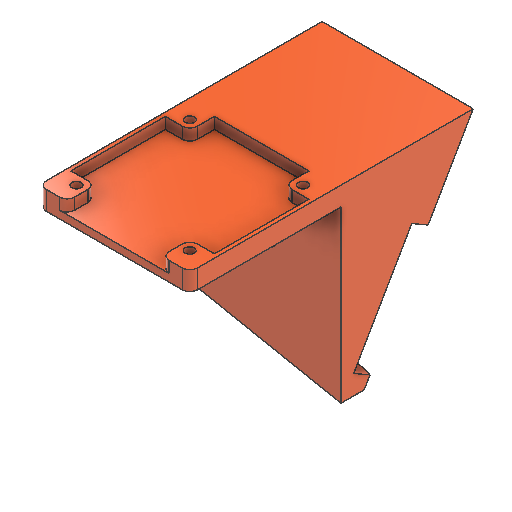
# Autodesk Inventor part: CameraMountM12v2
Saved by Autodesk Inventor 2025.2 (Build 292293000, 293)
## iProperties
Created: 2024-07-04
Part Number: CameraMountM12v2
Material: Generic
Document SubType Name: Modeling
Designer: rolan
Density: 1 g/cm^3
Appearance: Default
Author: rolan
Autodesk Inventor part; units mm, degrees
ref_plane "YZ Plane" through (0, 0, 0) normal (1, 0, 0) x (0, 1, 0)
ref_plane "XZ Plane" through (0, 0, 0) normal (0, 1, 0) x (-1, 0, 0)
sketch "Sketch1" plane through (0, 0, 0) normal (0, 1, 0) x (-1, 0, 0)
  line L0 (19, 19) -> (-19, 19) construction
  line L1 (-19, 19) -> (-19, -19) construction
  line L2 (-19, -19) -> (19, -19) construction
  line L3 (19, -19) -> (19, 19) construction
  line L4 (19, 19) -> (-19, -19) construction
  line L5 (-19, 19) -> (19, -19) construction
  circle A0 centre (15, -15) radius 1.25
  circle A1 centre (-15, -15) radius 1.25
  circle A2 centre (15, 15) radius 1.25
  circle A3 centre (-15, 15) radius 1.25
  line L6 (20, 20) -> (-20, 20)
  line L7 (-20, 20) -> (-20, -20)
  line L8 (-20, -20) -> (20, -20)
  line L9 (20, -20) -> (20, 20)
  line L10 (20, 20) -> (-20, -20) construction
  line L11 (-20, 20) -> (20, -20) construction
  point P0 (0, 0)
  dimension "d0" = 38
  dimension "d1" = 38
  dimension "d2" = 2.5
  dimension "d3" = 2.5
  dimension "d4" = 2.5
  dimension "d5" = 2.5
  dimension "d6" = 4
  dimension "d7" = 4
  dimension "d8" = 4
  dimension "d9" = 4
  dimension "d10" = 40
  dimension "d11" = 40
  constraints: 24 end point, 4 centre point, 4 midpoint, 4 parallel, 2 horizontal, 2 horizontal alignment, 2 perpendicular, 2 vertical alignment
  measures "d0" distance of L1.end L2.end
  measures "d1" distance of L0.end L1.end
  measures "d2" diameter of A1
  measures "d3" diameter of A0
  measures "d4" diameter of A2
  measures "d5" diameter of A3
  measures "d6" distance from line of L2 A0.centre
  measures "d7" distance from line of L3 A0.centre
  measures "d8" distance from line of L0 A3.centre
  measures "d9" distance from line of L1 A3.centre
  measures "d10" distance of L8.end L7.end
  measures "d11" distance of L7.end L6.end
extrude "Extrusion1" add sketch "Sketch1" along normal blind 5
sketch "Sketch2" plane through (0, 5, 0) normal (0, 1, 0) x (1, 0, 0)
  line L0 (-12.5, 19) -> (-12.5, 12.5)
  line L1 (-12.5, 12.5) -> (-19, 12.5)
  line L2 (-19, 12.5) -> (-19, -12.5)
  line L3 (-20, 20) -> (-20, -20) projected
  line L4 (-19, -12.5) -> (-12.5, -12.5)
  line L5 (-12.5, -12.5) -> (-12.5, -20)
  line L6 (-12.5, -20) -> (12.5, -20)
  line L7 (12.5, -20) -> (12.5, -12.5)
  line L8 (12.5, -12.5) -> (19, -12.5)
  line L9 (19, -12.5) -> (19, 12.5)
  line L10 (19, 12.5) -> (12.5, 12.5)
  line L11 (12.5, 12.5) -> (12.5, 19)
  line L12 (12.5, 19) -> (-12.5, 19)
  point P0 (0, 0)
  dimension "d14" = 25
  dimension "d15" = 6.5
  dimension "d16" = 25
  dimension "d17" = 7.5
  dimension "d18" = 6.5
  dimension "d19" = 6.5
  dimension "d20" = 25
  dimension "d21" = 6.5
  dimension "d22" = 12.5
  dimension "d24" = 12.5
  constraints: 24 end point, 8 perpendicular, 4 point on line, 1 parallel, 1 vertical
  measures "d14" distance of L0.start L11.end
  measures "d15" distance of L10.end L11.end
  measures "d16" distance of L8.end L9.end
  measures "d17" distance between parallel lines of L6 L8
  measures "d18" distance between parallel lines of L9 L11
  measures "d19" distance between parallel lines of L9 L7
  measures "d20" distance of L5.end L6.end
  measures "d21" distance between parallel lines of L2 L5
  measures "d22" horizontal distance of point (0, 0) L0.start
  measures "d24" horizontal distance of point (0, 0) L0.end
extrude "Extrusion2" cut sketch "Sketch2" against normal blind 3
sketch "Sketch3" plane through (0, 2, 0) normal (0, 1, 0) x (1, 0, 0)
  line L0 (12.5, -12.5) -> (12.5, -20) projected
  line L1 (-12.5, -20) -> (12.5, -20)
  line L2 (12.5, -20) -> (12.5, -16)
  line L3 (12.5, -16) -> (-12.5, -16)
  line L4 (-12.5, -16) -> (-12.5, -20)
  point P0 (0, 0)
  dimension "d27" = 4
  constraints: 8 end point, 2 parallel, 1 horizontal, 1 perpendicular, 1 point on line
  measures "d27" distance of L2.end L1.end
extrude "Extrusion3" cut sketch "Sketch3" against normal through all
fillet "Fillet1" radius 2 10 edges at (-20, 2.5, -20) (20, 2.5, -20) (-20, 2.5, 20) (20, 2.5, 20) (-12.5, 3.5, -12.5) (12.5, 3.5, -12.5) (12.5, 3.5, 12.5) (-12.5, 3.5, 12.5) (-12.5, 2.5, 20) (12.5, 2.5, 20)
sketch "Sketch4" plane through (0, 0, 0) normal (0, -1, 0) x (1, 0, 0)
  line L0 (-20, -17.5) -> (20, -17.5)
  line L1 (20, -17.5) -> (20, 17.5)
  line L2 (20, 17.5) -> (-20, 17.5)
  line L3 (-20, 17.5) -> (-20, -17.5)
  line L4 (-20, -17.5) -> (20, 17.5) construction
  line L5 (20, -17.5) -> (-20, 17.5) construction
  point P0 (0, 0)
  dimension "d31" = 40
  dimension "d32" = 35
  constraints: 12 end point, 2 midpoint, 2 parallel, 1 horizontal, 1 perpendicular
  measures "d31" distance of L2.end L1.end
  measures "d32" distance of L1.end L0.end
extrude "Extrusion4" add sketch "Sketch4" along normal blind 50
sketch "Sketch6" plane through (-20, 0, 17.5) normal (0, 0, 1) x (1, 0, 0)
  line L0 (40, 0) -> (40, -50) projected
  line L1 (40, -50) -> (0, -42.0435)
  line L2 (0, 0) -> (0, -50) projected
  line L3 (40, -50) -> (80.7836, -50) construction
  line L4 (0, -42.0435) -> (0, -50)
  line L5 (0, -50) -> (40, -50)
  point P0 (20, 0)
  dimension "d35" = 168.75
  constraints: 8 end point, 1 collinear, 1 equal length, 1 horizontal, 1 perpendicular, 1 point on line
  measures "d35" angle of L3 L1
extrude "Extrusion5" cut sketch "Sketch6" against normal through all
sketch "Sketch7" plane through (20, 0, 17.5) normal (1, 0, 0) x (0, 0, 1)
  line L0 (-35, 0) -> (-35, 50) projected
  line L1 (-35, 0) -> (-6.1325, 50)
  line L2 (-35, 50) -> (0, 50) projected
  line L3 (-35, 0) -> (22.735, 0) construction
  line L4 (-6.1325, 50) -> (-35, 50)
  line L5 (-35, 50) -> (-35, 0)
  point P0 (-17.5, 0)
  dimension "d38" = 120
  constraints: 8 end point, 2 horizontal, 1 equal length, 1 perpendicular, 1 point on line
  measures "d38" angle of L1 L3
extrude "Extrusion6" cut sketch "Sketch7" against normal through all
sketch "Sketch17" plane through (20, 0, -17.5) normal (0, -0.5, -0.8660254) x (-1, 0, 0)
  line L0 (40, -48.5477) -> (0, -57.735) construction
  line L1 (40, 0) -> (40, -48.5477) construction
  line L2 (0, 0) -> (40, 0) construction
  line L3 (0, -57.735) -> (0, 0) construction
  line L4 (0, -54.6569) -> (40, -45.4695) construction
  line L5 (0, -23.8758) -> (40, -14.6884) construction
  line L6 (0, -54.6569) -> (40, -45.4695)
  line L7 (40, -14.6884) -> (0, -23.8758)
  line L8 (0, -23.8758) -> (0, -54.6569)
  line L9 (40, -45.4695) -> (40, -14.6884)
  point P0 (20, -8.75)
  dimension "d60" = 30
  dimension "d61" = 3
  constraints: 12 end point, 4 point on line, 3 parallel, 1 collinear, 1 vertical
  measures "d60" distance between parallel lines of L4 L5
  measures "d61" distance between parallel lines of L4 L0
extrude "Extrusion9" cut sketch "Sketch17" against normal blind 5
sketch "Sketch18" plane through (20, 2.5, -13.1699) normal (0, -0.5, -0.8660254) x (-1, 0, 0)
  line L0 (40, -14.6884) -> (40, -45.4695) construction
  line L1 (0, -23.8758) -> (40, -14.6884) construction
  line L2 (0, -54.6569) -> (0, -23.8758) construction
  line L3 (40, -45.4695) -> (0, -54.6569) construction
  line L4 (0, -54.6569) -> (40, -14.6884) construction
  line L5 (0, -23.8758) -> (40, -45.4695) construction
  circle A0 centre (20, -34.6727) radius 2
  circle A1 centre (20, -34.6727) radius 4.6064
  point P0 (20, -8.75)
  dimension "d64" = 4
  constraints: 4 end point, 2 centre point, 1 coincident, 1 midpoint
  measures "d64" diameter of A0
extrude "Extrusion11" cut sketch "Sketch18" against normal through all contours A0
ref_plane "Work Plane3" through (20, 15.5, 9.3468) normal (0, -0.5, -0.8660254) x (-1, 0, 0)
sketch "Sketch20" plane through (20, 15.5, 9.3468) normal (0, -0.5, -0.8660254) x (-1, 0, 0)
  circle A0 centre (20, -34.6727) radius 2 projected
  circle A1 centre (20, -34.6727) radius 3.5
  point P0 (20, -8.75)
  dimension "d70" = 7
  constraints: 1 centre point, 1 coincident
  measures "d70" diameter of A1
extrude "Extrusion12" cut sketch "Sketch20" along normal blind 25
sketch "Sketch21" plane through (-20, 0, 17.5) normal (0, 0, 1) x (1, 0, 0)
  line L0 (0, 0) -> (40, 0)
  line L1 (40, 0) -> (40, -5)
  line L2 (40, -5) -> (0, -5)
  line L3 (0, -5) -> (0, 0)
  point P0 (20, 0)
  dimension "d73" = 5
  constraints: 8 end point, 2 parallel, 1 horizontal, 1 perpendicular
  measures "d73" distance of L0.end L1.end
extrude "Extrusion13" add sketch "Sketch21" along normal blind 40
sketch "Sketch22" plane through (20, 0, -18) normal (1, 0, 0) x (0, 0, -1)
  line L0 (2, 0) -> (0, 0) projected
  line L1 (-38, 5) -> (-36, 5) projected
  line L2 (2, 0) -> (-38, 0)
  line L3 (-38, 0) -> (-38, 5)
  line L4 (-38, 5) -> (2, 5)
  line L5 (2, 5) -> (2, 0)
  point P0 (-18, 0)
  constraints: 8 end point, 2 parallel, 1 horizontal, 1 perpendicular
extrude "Extrusion14" cut sketch "Sketch22" against normal through all
sketch "Sketch23" plane through (-20, 0, 57.5) normal (0, 1, 0) x (1, 0, 0)
  line L0 (40, 0) -> (0, 0) construction
  line L1 (20, 0) -> (20, 20) construction
  line L2 (39, 39) -> (1, 39) construction
  line L3 (1, 39) -> (1, 1) construction
  line L4 (1, 1) -> (39, 1) construction
  line L5 (39, 1) -> (39, 39) construction
  line L6 (39, 39) -> (1, 1) construction
  line L7 (1, 39) -> (39, 1) construction
  circle A0 centre (35, 5) radius 1.25
  line L8 (20, 20) -> (1, 20) construction
  circle A1 centre (5, 5) radius 1.25
  circle A2 centre (35, 35) radius 1.25
  circle A3 centre (5, 35) radius 1.25
  point P0 (20, 57.5)
  dimension "d78" = 20
  dimension "d79" = 38
  dimension "d80" = 38
  dimension "d81" = 4
  dimension "d82" = 2.5
  constraints: 16 end point, 4 centre point, 4 midpoint, 3 symmetric about line, 2 parallel, 1 horizontal, 1 perpendicular, 1 point on line, 1 vertical, 3 other
  measures "d78" distance of L1.start L1.end
  measures "d79" distance of L4.end L3.end
  measures "d80" distance of L3.end L2.end
  measures "d81" distance from line of L4 A0.centre
  measures "d82" diameter of A0
extrude "Extrusion15" cut sketch "Sketch23" against normal through all
sketch "Sketch24" plane through (-20, 0, 57.5) normal (0, 1, 0) x (1, 0, 0)
  line L0 (1, 7.5) -> (7.5, 7.5)
  line L1 (7.5, 7.5) -> (7.5, 0)
  line L2 (7.5, 0) -> (32.5, 0)
  line L3 (32.5, 0) -> (32.5, 7.5)
  line L4 (32.5, 7.5) -> (39, 7.5)
  line L5 (39, 7.5) -> (39, 32.5)
  line L6 (39, 32.5) -> (32.5, 32.5)
  line L7 (32.5, 32.5) -> (32.5, 39)
  line L8 (32.5, 39) -> (7.5, 39)
  line L9 (7.5, 39) -> (7.5, 32.5)
  line L10 (7.5, 32.5) -> (1, 32.5)
  line L11 (1, 32.5) -> (1, 7.5)
  line L12 (0, 0) -> (40, 0) construction
  line L13 (0, 75) -> (0, 0) projected
  point P0 (20, 57.5)
  point P1 (39, 20)
  point P2 (20, 39)
  dimension "d85" = 6.5
  dimension "d86" = 25
  dimension "d87" = 6.5
  dimension "d88" = 25
  dimension "d90" = 7.5
  dimension "d91" = 25
  dimension "d92" = 6.5
  dimension "d93" = 20
  dimension "d94" = 7.5
  dimension "d95" = 6.5
  dimension "d96" = 20
  constraints: 24 end point, 8 perpendicular, 3 horizontal, 2 midpoint, 2 point on line
  measures "d85" distance of L0.start L0.end
  measures "d86" distance of L1.end L2.end
  measures "d87" distance of L3.end L4.end
  measures "d88" distance of L7.end L8.end
  measures "d90" distance of L2.end L3.end
  measures "d91" distance of L4.end L5.end
  measures "d92" distance of L6.end L7.end
  measures "d93" distance from line of L12 point (39, 20)
  measures "d94" distance of L0.end L1.end
  measures "d95" distance of L8.end L9.end
  measures "d96" distance from line of L13 point (20, 39)
extrude "Extrusion16" cut sketch "Sketch24" against normal blind 3
fillet "Fillet2" radius 2 8 edges at (-12.5, -1.5, 50) (-12.5, -1.5, 25) (12.5, -1.5, 25) (12.5, -1.5, 50) (12.5, -1.5, 57.5) (-12.5, -1.5, 57.5) (20, -2.5, 57.5) (-20, -2.5, 57.5)
body "Solid1"
